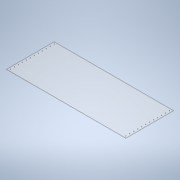
# Autodesk Inventor part: 12x30 Lexan
Saved by Autodesk Inventor 2020 (Build 240168000, 168)
## iProperties
Created: 2020-01-14
Part Number: 12x30 Lexan
Material: Polycarbonate, Clear
Document SubType Name: Modeling
Designer: aidan
Density: 1.2 g/cm^3
Appearance: Polycarbonate - Clear
Author: aidan
Autodesk Inventor part; units mm, degrees
ref_plane "YZ Plane" through (0, 0, 0) normal (1, 0, 0) x (0, 1, 0)
ref_plane "XZ Plane" through (0, 0, 0) normal (0, 1, 0) x (-1, 0, 0)
ref_plane "XY Plane" through (0, 0, 0) normal (0, 0, 1) x (1, 0, 0)
sketch "Sketch1" plane through (0, 0, 0) normal (0, 1, 0) x (-1, 0, 0)
  line L0 (374.9202, 41.3426) -> (-387.0798, 41.3426)
  line L1 (-387.0798, 41.3426) -> (-387.0798, -263.4574)
  line L2 (-387.0798, -263.4574) -> (374.9202, -263.4574)
  line L3 (374.9202, -263.4574) -> (374.9202, 41.3426)
  point P0 (0, 0)
  dimension "d0" = 304.8
  dimension "d1" = 762
  constraints: 8 end point, 2 parallel, 1 horizontal, 1 perpendicular
  measures "d0" distance of L2.end L0.start
  measures "d1" distance of L1.end L2.end
extrude "Extrusion1" add sketch "Sketch1" along normal blind 2.9972
sketch "Sketch2" plane through (0, 2.9972, 0) normal (0, 1, 0) x (1, 0, 0)
  circle A0 centre (-362.2202, -28.6426) radius 1.7272
  line L0 (-374.9202, 263.4574) -> (-374.9202, -41.3426) projected
  line L1 (-374.9202, -41.3426) -> (387.0798, -41.3426) projected
  point P0 (0, 0)
  dimension "d4" = 3.4544
  dimension "d5" = 12.7
  dimension "d6" = 12.7
  constraints: 1 centre point
  measures "d4" diameter of A0
  measures "d5" distance from line of L0 A0.centre
  measures "d6" distance from line of L1 A0.centre
extrude "Extrusion2" cut sketch "Sketch2" against normal through all
pattern_linear "Rectangular Pattern1" count 12 spacing 25.4 along (0, 0, -1) count 2 spacing 736.6 along (1, 0, 0) of "Extrusion2"
body "Solid1"
